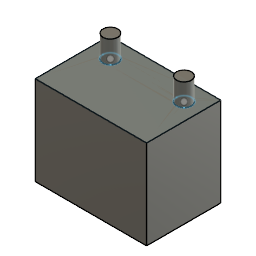
battery (Autodesk Fusion 360 design; units mm, degrees)
part number: 2026-02-08-14-35-29-310
Autodesk Fusion 360 part; units mm, degrees
sketch "Sketch1" plane through (0, 0, 0) normal (0, 1, 0) x (1, 0, 0)
  line L0 (-31.3279, 23.8092) -> (159.1721, 23.8092)
  line L1 (159.1721, 23.8092) -> (159.1721, -103.1908)
  line L2 (159.1721, -103.1908) -> (-31.3279, -103.1908)
  line L3 (-31.3279, -103.1908) -> (-31.3279, 23.8092)
  dimension "d1" = 190.5
  dimension "d2" = 127
  constraint horizontal L0
  constraint vertical L1
  constraint horizontal L2
  constraint vertical L3
  measures "d1" distance of L0.start L0.end
  measures "d2" distance of L0.start L2.end
extrude "Extrude1" add sketch "Sketch1" along normal blind 152.4
sketch "Sketch2" plane through (0, 152.4, 0) normal (0, 1, 0) x (-1, 0, 0)
  line L0 (31.3279, 103.1908) -> (-159.1721, 103.1908)
  line L1 (-159.1721, 103.1908) -> (-159.1721, -23.8092)
  line L2 (-159.1721, -23.8092) -> (31.3279, -23.8092)
  line L3 (31.3279, -23.8092) -> (31.3279, 103.1908)
  circle A0 centre (-3.5457, 9.4553) radius 12.7
  circle A1 centre (-130, 10) radius 12.7
  dimension "d5" = 25.4
  dimension "d6" = 25.4
  measures "d5" diameter of A0
  measures "d6" diameter of A1
extrude "Extrude2" add sketch "Sketch2" along normal blind 38.1 contours A0
extrude "Extrude3" add sketch "Sketch2" along normal blind 38.1 contours A1
